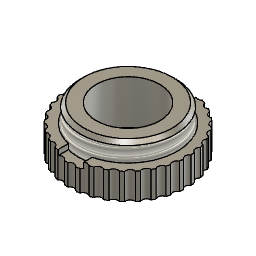
Eurorack Jack Top (Autodesk Fusion 360 design; units mm, degrees)
Autodesk Fusion 360 part; units mm, degrees
note: some values were not read from the file. Chosen so that the rebuilt part matches the saved one: how an offset face is resized. Set by a fixed rule: which sketch regions a step uses; which face or edge a step refers to.
sketch "Sketch1" plane through (0, 0, 0) normal (0, 1, 0) x (1, 0, 0)
  circle A0 centre (0, 0) radius 1.8
  circle A1 centre (0, 0) radius 2.8
  circle A2 centre (0, 0) radius 3.375
  line L0 (0.675, -4.2965) -> (-0.675, -4.2965)
  line L1 (-0.675, -4.2965) -> (-0.675, 4.2965)
  line L2 (-0.675, 4.2965) -> (0.675, 4.2965)
  line L3 (0.675, 4.2965) -> (0.675, -4.2965)
  line L4 (0.675, -4.2965) -> (-0.675, 4.2965) construction
  line L5 (-0.675, -4.2965) -> (0.675, 4.2965) construction
  circle A3 centre (3.5, 0) radius 0.25
  circle A4 centre (3.4368, 0.6624) radius 0.25
  circle A5 centre (3.2493, 1.3008) radius 0.25
  circle A6 centre (2.9444, 1.8922) radius 0.25
  circle A7 centre (2.5331, 2.4153) radius 0.25
  circle A8 centre (2.0302, 2.851) radius 0.25
  circle A9 centre (1.454, 3.1837) radius 0.25
  circle A10 centre (0.8252, 3.4013) radius 0.25
  circle A11 centre (0.1665, 3.496) radius 0.25
  circle A12 centre (-0.4981, 3.4644) radius 0.25
  circle A13 centre (-1.1447, 3.3075) radius 0.25
  circle A14 centre (-1.75, 3.0311) radius 0.25
  circle A15 centre (-2.292, 2.6451) radius 0.25
  circle A16 centre (-2.7512, 2.1636) radius 0.25
  circle A17 centre (-3.1109, 1.6038) radius 0.25
  circle A18 centre (-3.3582, 0.9861) radius 0.25
  circle A19 centre (-3.4842, 0.3327) radius 0.25
  circle A20 centre (-3.4842, -0.3327) radius 0.25
  circle A21 centre (-3.3582, -0.9861) radius 0.25
  circle A22 centre (-3.1109, -1.6038) radius 0.25
  circle A23 centre (-2.7512, -2.1636) radius 0.25
  circle A24 centre (-2.292, -2.6451) radius 0.25
  circle A25 centre (-1.75, -3.0311) radius 0.25
  circle A26 centre (-1.1447, -3.3075) radius 0.25
  circle A27 centre (-0.4981, -3.4644) radius 0.25
  circle A28 centre (0.1665, -3.496) radius 0.25
  circle A29 centre (0.8252, -3.4013) radius 0.25
  circle A30 centre (1.454, -3.1837) radius 0.25
  circle A31 centre (2.0302, -2.851) radius 0.25
  circle A32 centre (2.5331, -2.4153) radius 0.25
  circle A33 centre (2.9444, -1.8922) radius 0.25
  circle A34 centre (3.2493, -1.3008) radius 0.25
  circle A35 centre (3.4368, -0.6624) radius 0.25
  dimension "d1" = 3.6
  dimension "d2" = 5.6
  dimension "d3" = 6.75
  dimension "d4" = 1.35
  dimension "d5" = 0.5
  dimension "d7" = 360
  constraint coincident A0.centre A1.centre
  constraint concentric A1 A2
  constraint horizontal L0
  constraint perpendicular L0 L1
  constraint parallel L0 L2
  constraint parallel L1 L3
  constraint coincident L4 A0.centre
  constraint coincident L5 A0.centre
  measures "d1" diameter of A0
  measures "d2" diameter of A1
  measures "d3" diameter of A2
  measures "d4" distance of L1.end L2.end
  measures "d5" diameter of A3
extrude "Extrude1" add sketch "Sketch1" along normal blind 2.5 contours A0 A1 L3 | A0 A1 L1 L3 | A0 A1 L1 L3 | A0 A1 L1 makes body 1
extrude "Extrude2" add sketch "Sketch1" along normal blind 1.2 separate body contours A1 A2 L1 L3 A10 A11 A12 | A1 A2 L1 L3 A27 A28 A29 makes body 2 at (0.5642, 0.8, 2.7426) makes body 3 at (-0.5642, 0.8, -2.7426)
extrude "Extrude3" add sketch "Sketch1" along normal blind 1.5 contours A1 A2 L3 A3 A4 A5 A6 A7 A8 A9 A10 A29 A30 A31 A32 A33 A34 A35 | A1 A2 L1 A12 A13 A14 A15 A16 A17 A18 A19 A20 A21 A22 A23 A24 A25 A26 A27 bodies 2 3
thread "Thread1" "ISO Metric profile 5.5 M5.5x0.5 6g" major diameter 5.427 minor diameter 4.848 pitch 0.5 angle 60 resizes the face on face at (0.5642, 1.6667, 2.7426) on bodies 1
chamfer "Chamfer1" distance 0.2 angle 45 1 edges at (-2.5299, 2.5, 0.9812) on bodies 1
